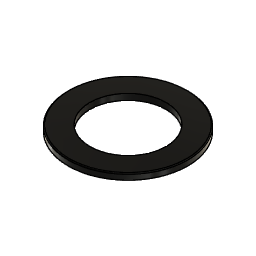
camera-and-led-ring-mount-by-3dengelen (Autodesk Fusion 360 archive; units mm, degrees)
design "Surround"
Autodesk Fusion 360 part; units mm, degrees
sketch "Sketch1" plane through (0, 0, 0) normal (0, 0, 1) x (1, 0, 0)
  circle A0 centre (0, 0) radius 345
  circle A1 centre (0, 0) radius 220
  dimension "d1" = 690
  dimension "d2" = 440
  constraint coincident A0.centre A1.centre
  measures "d1" diameter of A0
  measures "d2" diameter of A1
extrude "Extrude1" add sketch "Sketch1" along normal blind 35
fillet "Fillet1" radius 5 1 edges at (-321.6529, -124.7573, 35)

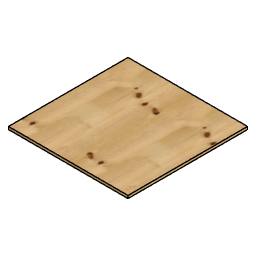
design "BackPlate"
Autodesk Fusion 360 part; units mm, degrees
sketch "Sketch1" plane through (0, 0, 0) normal (0, 0, 1) x (1, 0, 0)
  line L0 (400, -400) -> (-400, -400)
  line L1 (-400, -400) -> (-400, 400)
  line L2 (-400, 400) -> (400, 400)
  line L3 (400, 400) -> (400, -400)
  line L4 (400, -400) -> (-400, 400) construction
  line L5 (-400, -400) -> (400, 400) construction
  dimension "d1" = 800
  dimension "d2" = 800
  constraint horizontal L0
  constraint perpendicular L0 L1
  constraint parallel L0 L2
  constraint parallel L1 L3
  constraint coincident L4 origin
  constraint coincident L5 origin
  measures "d1" distance of L1.end L2.end
  measures "d2" distance of L0.end L1.end
extrude "Extrude1" add sketch "Sketch1" along normal blind 18
